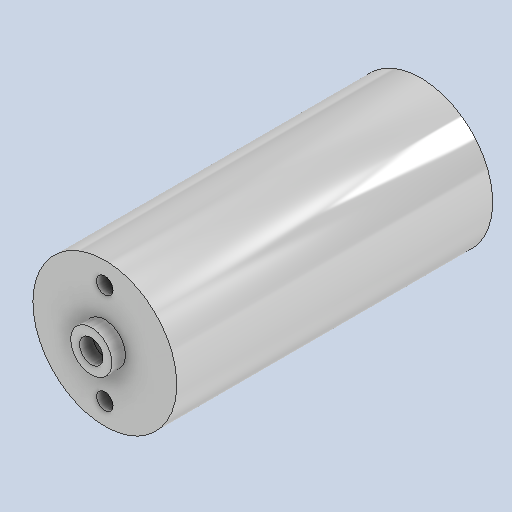
# Autodesk Inventor part: 馬達
Saved by Autodesk Inventor 2024 (Build 280153000, 153)
## iProperties
Created: 2024-03-30
Part Number: 馬達
Material: 鋁合金 6061
Document SubType Name: Modeling
Designer: USER
Density: 2.7 g/cm^3
Appearance: 鋁 - 拋光
Author: USER
Autodesk Inventor part; units mm, degrees
ref_plane "YZ Plane" through (0, 0, 0) normal (1, 0, 0) x (0, 1, 0)
ref_plane "XZ Plane" through (0, 0, 0) normal (0, 1, 0) x (-1, 0, 0)
ref_plane "XY Plane" through (0, 0, 0) normal (0, 0, 1) x (1, 0, 0)
sketch "草圖1" plane through (0, 0, 0) normal (0, 1, 0) x (-1, 0, 0)
  line L0 (12.2, 0) -> (-12.2, 0)
  line L1 (-12.2, 0) -> (-12.2, -53.6)
  line L2 (-12.2, -53.6) -> (12.2, -53.6)
  line L3 (12.2, -53.6) -> (12.2, 0)
  line L4 (2, 0) -> (-2, 0)
  line L5 (-2, 0) -> (-2, 12)
  line L6 (-2, 12) -> (2, 12)
  line L7 (2, 12) -> (2, 0)
  line L8 (3.5, 0) -> (-3.5, 0)
  line L9 (-3.5, 0) -> (-3.5, 2.3)
  line L10 (-3.5, 2.3) -> (3.5, 2.3)
  line L11 (3.5, 2.3) -> (3.5, 0)
  line L12 (2, 4) -> (-2, 4)
  line L13 (8.5, 0) -> (8.5, -53.6)
  line L14 (-8.5, 0) -> (-8.5, -53.6)
  line L15 (0, 0) -> (0, -53.6)
  line L16 (0, 0) -> (0, 12)
  point P0 (-8.5, -26.8)
  point P1 (0, 2.3)
  point P2 (2, 2.3)
  dimension "d1" = 8
  dimension "d2" = 9.7
  dimension "d4" = 17
  dimension "d5" = 24.4
  dimension "d6" = 53.6
  dimension "d7" = 3.7
  dimension "d8" = 4
  dimension "d9" = 7
  dimension "d10" = 2.3
  constraints: 34 end point, 8 point on line, 6 parallel, 6 perpendicular, 5 midpoint, 3 horizontal, 2 vertical alignment, 1 coincident, 1 vertical
  measures "d1" distance of L6.end L12.start
  measures "d2" vertical distance of L9.end L5.end
  measures "d4" distance from line of point (-8.5, -26.8) L13
  measures "d5" distance of L1.end L2.end
  measures "d6" distance of L0.end L1.end
  measures "d7" distance of L2.end L13.end
  measures "d8" distance of L5.end L6.end
  measures "d9" distance of L9.end L10.end
  measures "d10" distance of L8.start L10.end
revolve "迴轉1" add sketch "草圖1" angle 360 about axis through (0, 0, 0) along (0, 0, -1) contours L3 L2 L13 L0 | L13 L2 L15 L0 | L0 L7 L10 L11
sketch "草圖4" plane through (0, 0, 0) normal (0, 0, 1) x (1, 0, 0)
  circle A0 centre (0, 0) radius 8.5
  circle A1 centre (0, 8.5) radius 1.4
  circle A2 centre (0, -8.5) radius 1.4
  dimension "d21" = 17
  dimension "d22" = 2.8
  dimension "d23" = 2.8
  constraints: 3 centre point, 2 point on circle, 2 vertical alignment, 1 coincident
  measures "d21" diameter of A0
  measures "d22" diameter of A1
  measures "d23" diameter of A2
extrude "擠出3" cut sketch "草圖4" against normal blind 3 contours A1 A0 | A0 A1 | A2 A0 | A0 A2
